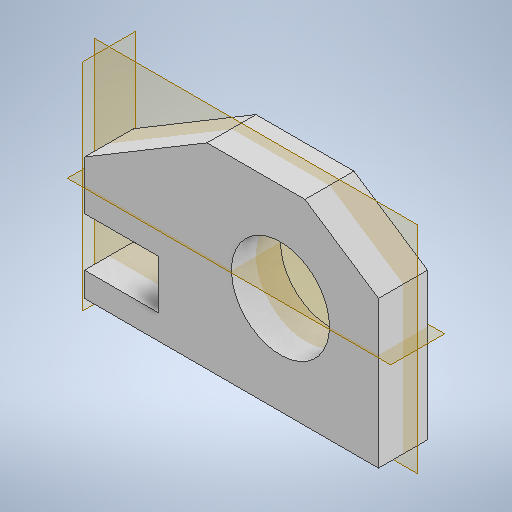
# Autodesk Inventor part: chap2ex1
Saved by Autodesk Inventor 2025.2 (Build 292293000, 293)
## iProperties
Created: 2025-01-31
Part Number: chap2ex1
Material: Generic
Document SubType Name: Modeling
Designer: Moofin
Density: 1 g/cm^3
Appearance: Default
Author: Moofin
Autodesk Inventor part; units mm, degrees
sketch "Sketch1" plane through (0, 0, 0) normal (0, 0, 1) x (1, 0, 0)
  line L0 (0, 25.4) -> (76.2, 25.4)
  line L1 (76.2, 25.4) -> (76.2, -25.4)
  line L2 (76.2, -25.4) -> (0, -25.4)
  line L3 (0, -25.4) -> (0, 25.4)
  line L4 (-15.24, 0) -> (91.44, 0) projected
  line L5 (0, 35.56) -> (0, -35.56) projected
  point P0 (0, 0)
  dimension "d0" = 50.8
  dimension "d1" = 76.2
  dimension "d2" = 25.4
  dimension "d3" = 0
  constraints: 8 end point, 2 parallel, 1 horizontal, 1 perpendicular
  measures "d0" distance of L2.end L0.start
  measures "d1" distance of L0.start L0.end
  measures "d2" distance between parallel lines of L4 L0
  measures "d3" distance between parallel lines of L5 L3
extrude "Extrusion1" add sketch "Sketch1" along normal mid plane 12.7
sketch "Sketch2" plane through (0, 0, 6.35) normal (0, 0, 1) x (1, 0, 0)
  circle A0 centre (50.8, 0) radius 12.7
  line L0 (76.2, -25.4) -> (76.2, 25.4) projected
  line L1 (0, -25.4) -> (76.2, -25.4) projected
  point P0 (0, 0)
  dimension "d6" = 25.4
  dimension "d7" = 25.4
  dimension "d8" = 25.4
  constraints: 1 centre point
  measures "d6" distance from line of L0 A0.centre
  measures "d7" distance from line of L1 A0.centre
  measures "d8" diameter of A0
extrude "Extrusion2" cut sketch "Sketch2" against normal up to surface (12.7 mm away)
sketch "Sketch3" plane through (0, 0, 6.35) normal (0, 0, 1) x (1, 0, 0)
  line L0 (0, -25.4) -> (0, 25.4) projected
  line L1 (0, -6.35) -> (19.05, -6.35)
  line L2 (19.05, -6.35) -> (19.05, -19.05)
  line L3 (19.05, -19.05) -> (0, -19.05)
  line L4 (0, -25.4) -> (76.2, -25.4) projected
  point P0 (0, 0)
  dimension "d11" = 12.7
  dimension "d12" = 19.05
  dimension "d13" = 6.35
  constraints: 6 end point, 2 point on line, 1 horizontal, 1 parallel, 1 perpendicular
  measures "d11" distance between parallel lines of L3 L1
  measures "d12" distance between parallel lines of L0 L2
  measures "d13" distance between parallel lines of L4 L3
extrude "Extrusion3" cut sketch "Sketch3" against normal up to surface (12.7 mm away)
chamfer "Chamfer1" distance 12.7 distance2 19.05 1 edges at (76.2, 25.4, 0) measured on face at (76.2, 8.4667, 2.1167)
chamfer "Chamfer2" distance 31.75 distance2 19.05 1 edges at (0, 25.4, 0) measured on face at (19.05, 25.4, 2.1167)
equation "\"d2\" = 0.5 * d0"
body "Solid1"
